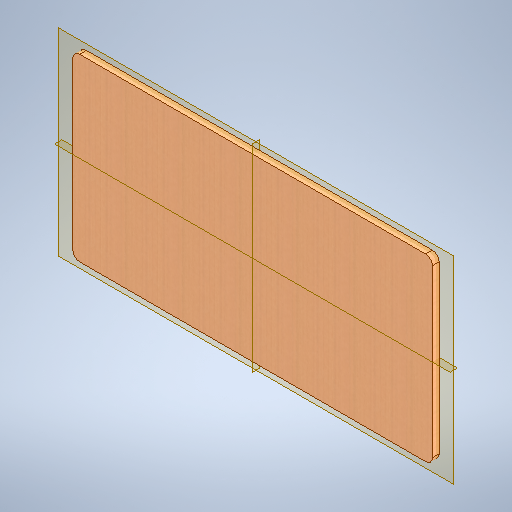
# Autodesk Inventor part: Sessao7_02_04_2025_999_0001
Saved by Autodesk Inventor 2025.2 (Build 292293000, 293)
## iProperties
Created: 2025-04-02
Part Number: Sessao7_02_04_2025_999_0001
Material: Madeira (Cerejeira)
Document SubType Name: Modeling
Designer: lucas
Density: 0.63 g/cm^3
Appearance: Cerejeira - Natural com pouco brilho
Author: lucas
Autodesk Inventor part; units mm, degrees
sketch "Esboço1" plane through (0, 0, 0) normal (0, 0, 1) x (1, 0, 0)
  line L0 (-800, -400) -> (800, -400)
  line L1 (800, -400) -> (800, 400)
  line L2 (800, 400) -> (-800, 400)
  line L3 (-800, 400) -> (-800, -400)
  line L4 (-800, -400) -> (800, 400) construction
  line L5 (800, -400) -> (-800, 400) construction
  point P0 (0, 0)
  dimension "d0" = 1600
  dimension "d1" = 800
  constraints: 12 end point, 2 midpoint, 2 parallel, 1 horizontal, 1 perpendicular
  measures "d0" distance of L1.end L2.end
  measures "d1" distance of L0.end L1.end
extrude "Extrusão1" add sketch "Esboço1" along normal mid plane 30
fillet "Arredondamento1" radius 30 1 edges at (-800, 400, 0)
fillet "Arredondamento2" radius 30 1 edges at (800, 400, 0)
fillet "Arredondamento3" radius 30 1 edges at (800, -400, 0)
fillet "Arredondamento4" radius 30 1 edges at (-800, -400, 0)
sketch "Esboço3" plane through (0, 0, -15) normal (0, 0, -1) x (-1, 0, 0)
  circle A0 centre (-750, 350) radius 35.4
  circle A1 centre (-750, 350) radius 17.1
  point P0 (0, 0)
  dimension "d9" = 70.8
  dimension "d10" = 350
  dimension "d11" = 750
  dimension "d13" = 34.2
  constraints: 2 centre point, 1 coincident
  measures "d9" diameter of A0
  measures "d10" vertical distance of point (0, 0) A0.centre
  measures "d11" horizontal distance of point (0, 0) A0.centre
  measures "d13" diameter of A1
extrude "Extrusão2" cut sketch "Esboço3" against normal blind 15
mirror "Espelhar1" about plane through (0, 0, 0) normal (1, 0, 0) of "Extrusão2"
mirror "Espelhar2" about plane through (0, 0, 0) normal (0, 1, 0) of "Extrusão2", "Espelhar1"
